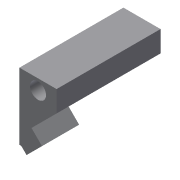
# Autodesk Inventor part: sampleHolder_v3
Saved by Autodesk Inventor 2013 (Build 170138000, 138)
## iProperties
Created: 2014-12-18
Part Number: sampleHolder_v3
Material: Generic
Document SubType Name: Modeling
Designer: 120pa
Density: 1 g/cm^3
Author: 120pa
Autodesk Inventor part; units mm, degrees
ref_plane "YZ Plane" through (0, 0, 0) normal (1, 0, 0) x (0, 1, 0)
ref_plane "XZ Plane" through (0, 0, 0) normal (0, 1, 0) x (-1, 0, 0)
ref_plane "XY Plane" through (0, 0, 0) normal (0, 0, 1) x (1, 0, 0)
sketch "Sketch1" plane through (0, 0, 0) normal (0, 1, 0) x (-1, 0, 0)
  line L0 (0, -5.6886) -> (6.7556, -12.4442)
  line L1 (6.7556, -12.4442) -> (5.3414, -13.8584)
  line L2 (9.5, -18.017) -> (5.3414, -13.8584)
  line L3 (10, -18.017) -> (9.5, -18.017)
  line L4 (10, -18.017) -> (10, 0)
  line L5 (0, 0) -> (10, 0)
  line L6 (0, 0) -> (0, -5.6886)
  circle A0 centre (5, -2.8443) radius 1.339
  constraints: 14 end point, 1 centre point
extrude "Extrusion1" add sketch "Sketch1" along normal blind 10
sketch "Sketch2" plane through (0, 10, 0) normal (0, 1, 0) x (1, 0, 0)
  line L0 (0, 5.6886) -> (-10, 5.6886)
  line L1 (-10, 5.6886) -> (-10, 0)
  line L2 (-10, 0) -> (0, 0)
  line L3 (0, 0) -> (0, 5.6886)
  constraints: 8 end point
extrude "Extrusion2" add sketch "Sketch2" along normal blind 20
sketch "Sketch3" plane through (0, 0, 0) normal (0, -1, 0) x (1, 0, 0)
  circle A0 centre (-5, -2.8443) radius 1.339 projected
hole "Hole1" at (-5, 0, -2.8443) direction (0, 1, 0) diameter 4.318 depth 31 tip angle 118
sketch "Sketch4" plane through (-9.5, 0, -18.017) normal (0.7071, 0, -0.7071) x (-0.7071, 0, -0.7071)
  circle A0 centre (-2.9406, 5) radius 2.55
  point P0 (-19.4575, 0)
  dimension "d11" = 5.1
  constraints: 1 centre point
  measures "d11" diameter of A0
extrude "Extrusion3" cut sketch "Sketch4" against normal blind 0.1
sketch "Sketch6" plane through (-9.5, 0, -18.017) normal (0.7071, 0, -0.7071) x (-0.7071, 0, -0.7071)
  circle A0 centre (-2.9406, 5) radius 2.55 projected
  line L0 (-5.8811, 0) -> (0, 0) projected
  line L1 (0, 0) -> (0, 10) projected
  line L2 (-5.8811, 10) -> (0, 10) projected
  line L3 (-5.8811, 0) -> (-5.8811, 10) projected
  point P0 (-19.4575, 0)
sketch "Sketch8" plane through (0, 30, 0) normal (0, 1, 0) x (1, 0, 0)
  circle A0 centre (-5, 2.8443) radius 2.159 projected
  line L0 (0, 5.6886) -> (-10, 5.6886) projected
  line L1 (-10, 5.6886) -> (-10, 0) projected
  line L2 (-10, 0) -> (0, 0) projected
  line L3 (0, 0) -> (0, 5.6886) projected
extrude "Extrusion5" cut sketch "Sketch8" against normal blind 2
extrude "Extrusion6" add sketch "Sketch6" along normal blind 2
sketch "Sketch9" plane through (-8.0858, 0, -19.4312) normal (0.7071, 0, -0.7071) x (-0.7071, 0, -0.7071)
  line L0 (-4.9902, 1.1733) -> (-0.8909, 1.1733)
  line L1 (-0.8909, 1.1733) -> (-0.8909, 8.8267)
  line L2 (-0.8909, 8.8267) -> (-4.9902, 8.8267)
  line L3 (-4.9902, 8.8267) -> (-4.9902, 1.1733)
  line L4 (-4.9902, 1.1733) -> (-0.8909, 8.8267) construction
  line L5 (-0.8909, 1.1733) -> (-4.9902, 8.8267) construction
  point P0 (-19.4575, 0)
  point P1 (-2.9406, 5)
  constraints: 12 end point, 2 midpoint
extrude "Extrusion7" cut sketch "Sketch9" against normal blind 0.2
sketch "Sketch10" plane through (-8.2272, 0, -19.2898) normal (0.7071, 0, -0.7071) x (-0.7071, 0, -0.7071)
  line L0 (-4.9902, 8.3098) -> (-0.8909, 8.3098)
  line L1 (-0.8909, 8.3098) -> (-0.8909, 8.8267)
  line L2 (-0.8909, 8.8267) -> (-4.9902, 8.8267)
  line L3 (-4.9902, 8.8267) -> (-4.9902, 8.3098)
  point P0 (-19.4575, 0)
  constraints: 8 end point
extrude "Extrusion8" cut sketch "Sketch10" against normal blind 0.3
sketch "Sketch11" plane through (-8.2272, 0, -19.2898) normal (0.7071, 0, -0.7071) x (-0.7071, 0, -0.7071)
  line L0 (-4.9902, 1.1733) -> (-0.8909, 1.1733)
  line L1 (-0.8909, 1.1733) -> (-0.8909, 1.613)
  line L2 (-0.8909, 1.613) -> (-4.9902, 1.613)
  line L3 (-4.9902, 1.613) -> (-4.9902, 1.1733)
  point P0 (-19.4575, 0)
  constraints: 8 end point
extrude "Extrusion9" cut sketch "Sketch11" against normal blind 0.3
body "Solid1"
